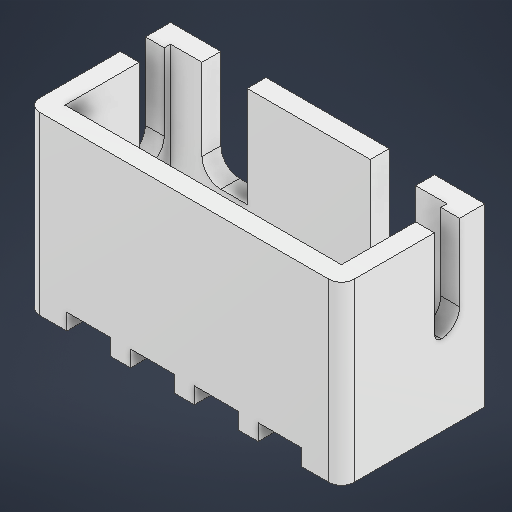
# Autodesk Inventor part: 4pin_head
Saved by Autodesk Inventor 2026 (Build 300175000, 175)
## iProperties
Created: 2025-04-18
Part Number: 4pin_head
Material: ABS Plastic
Document SubType Name: Modeling
Designer: ct_vi
Density: 1.06 g/cm^3
Appearance: Smooth - White
Author: ct_vi
Autodesk Inventor part; units mm, degrees
ref_plane "YZ Plane" through (0, 0, 0) normal (1, 0, 0) x (0, 1, 0)
ref_plane "XZ Plane" through (0, 0, 0) normal (0, 1, 0) x (-1, 0, 0)
ref_plane "XY Plane" through (0, 0, 0) normal (0, 0, 1) x (1, 0, 0)
sketch "Sketch1" plane through (0, 0, 0) normal (0, 1, 0) x (-1, 0, 0)
  line L0 (-10.6149, 17.6203) -> (28.5511, 17.6203) construction
  line L1 (28.5511, 17.6203) -> (28.5511, -21.5457) construction
  line L2 (28.5511, -21.5457) -> (-10.6149, -21.5457) construction
  line L3 (-10.6149, -21.5457) -> (-10.6149, 17.6203) construction
  line L4 (6.25, 2.85) -> (-6.25, 2.85)
  line L5 (-6.25, 2.85) -> (-6.25, -2.85)
  line L6 (-6.25, -2.85) -> (6.25, -2.85)
  line L7 (6.25, -2.85) -> (6.25, 2.85)
  line L8 (6.25, 2.85) -> (-6.25, -2.85) construction
  line L9 (-6.25, 2.85) -> (6.25, -2.85) construction
  line L10 (0, -2.85) -> (0, -0.85)
  line L11 (0, -0.85) -> (0, -0.54)
  line L12 (-0.96, -0.23) -> (-1.58, -0.23)
  line L13 (-1.58, -0.23) -> (-1.58, -0.85)
  line L14 (-1.58, -0.85) -> (-0.96, -0.85)
  line L15 (-0.96, -0.85) -> (-0.96, -0.23)
  line L16 (-0.96, -0.23) -> (-1.58, -0.85) construction
  line L17 (-1.58, -0.23) -> (-0.96, -0.85) construction
  line L18 (0.96, -0.23) -> (1.58, -0.23)
  line L19 (1.58, -0.23) -> (1.58, -0.85)
  line L20 (1.58, -0.85) -> (0.96, -0.85)
  line L21 (0.96, -0.85) -> (0.96, -0.23)
  line L22 (0.96, -0.23) -> (1.58, -0.85) construction
  line L23 (1.58, -0.23) -> (0.96, -0.85) construction
  line L24 (3.5, -0.23) -> (4.12, -0.23)
  line L25 (4.12, -0.23) -> (4.12, -0.85)
  line L26 (4.12, -0.85) -> (3.5, -0.85)
  line L27 (3.5, -0.85) -> (3.5, -0.23)
  line L28 (3.5, -0.23) -> (4.12, -0.85) construction
  line L29 (4.12, -0.23) -> (3.5, -0.85) construction
  line L30 (-3.5, -0.23) -> (-4.12, -0.23)
  line L31 (-4.12, -0.23) -> (-4.12, -0.85)
  line L32 (-4.12, -0.85) -> (-3.5, -0.85)
  line L33 (-3.5, -0.85) -> (-3.5, -0.23)
  line L34 (-3.5, -0.23) -> (-4.12, -0.85) construction
  line L35 (-4.12, -0.23) -> (-3.5, -0.85) construction
  line L36 (1.27, -0.54) -> (0, -0.54)
  line L37 (0, -0.54) -> (-1.27, -0.54)
  line L38 (-1.27, -0.54) -> (-3.81, -0.54)
  line L39 (-5.5, -2.1) -> (5.5, -2.1)
  line L40 (5.5, -2.1) -> (5.5, 2.1)
  line L41 (5.5, 2.1) -> (-5.5, 2.1)
  line L42 (-5.5, 2.1) -> (-5.5, -2.1)
  line L43 (-5.5, -2.1) -> (5.5, 2.1) construction
  line L44 (5.5, -2.1) -> (-5.5, 2.1) construction
  line L45 (0, -0.54) -> (0, -0.04)
  line L46 (-5.5, 0.2067) -> (5.5, 0.2067)
  line L47 (-5.5, -1.1747) -> (5.5, -1.1747)
  line L48 (5.5, -1.1747) -> (5.5, 0.2067)
  line L49 (-5.5, 0.2067) -> (-5.5, -1.1747)
  point P0 (0, 0)
  dimension "d11" = 12.5
  dimension "d12" = 5.7
  dimension "d43" = 2
  dimension "d44" = 0.31
  dimension "d57" = 0.62
  dimension "d58" = 0.62
  dimension "d59" = 2.54
  dimension "d66" = 11
  dimension "d68" = 0.75
  dimension "d72" = 0.5
  constraints: 92 end point, 14 parallel, 9 midpoint, 8 horizontal, 7 perpendicular, 3 point on line, 2 vertical, 2 other
  measures "d11" distance of L6.end L5.end
  measures "d12" distance of L5.end L4.end
  measures "d43" distance of L10.start L10.end
  measures "d44" distance of L10.end L11.end
  measures "d57" distance of L32.end L31.end
  measures "d58" distance of L31.end L30.end
  measures "d59" distance of L37.end L38.end
  measures "d66" distance of L41.end L40.end
  measures "d68" distance between parallel lines of L41 L4
  measures "d72" distance of L11.end L45.end
extrude "Extrusion1" add sketch "Sketch1" along normal blind 7 contours L7 L6 L5 L4
fillet "Fillet1" radius 0.5 2 edges at (6.25, 3.5, 2.85) (-6.25, 3.5, 2.85)
sketch "Sketch2" plane through (6.25, 0, -2.85) normal (0, 0, -1) x (-1, 0, 0)
  line L0 (-3.8851, 33.7763) -> (36.1854, 33.7763) construction
  line L1 (36.1854, 33.7763) -> (36.1854, -6.2941) construction
  line L2 (36.1854, -6.2941) -> (-3.8851, -6.2941) construction
  line L3 (-3.8851, -6.2941) -> (-3.8851, 33.7763) construction
  line L4 (6.25, 0) -> (6.25, 0.65)
  line L5 (0, 0) -> (12.5, 0) projected
  line L6 (5.85, 0) -> (6.65, 0)
  line L7 (6.25, 0.65) -> (3.71, 0.65)
  line L8 (3.71, 0.65) -> (4.11, 0.65)
  line L9 (4.11, 0.65) -> (3.31, 0.65)
  line L10 (3.31, 0.65) -> (3.31, 0)
  line L11 (3.31, 0) -> (4.11, 0)
  line L12 (4.11, 0) -> (4.11, 0.65)
  line L13 (6.25, 0.65) -> (8.79, 0.65)
  line L14 (8.79, 0.65) -> (8.39, 0.65)
  line L15 (8.39, 0.65) -> (9.19, 0.65)
  line L16 (9.19, 0.65) -> (9.19, 0)
  line L17 (9.19, 0) -> (8.39, 0)
  line L18 (8.39, 0) -> (8.39, 0.65)
  line L19 (6.25, 0.65) -> (6.65, 0.65)
  line L20 (6.65, 0.65) -> (5.85, 0.65)
  line L21 (5.85, 0.65) -> (5.85, 0)
  line L22 (5.85, 0) -> (6.65, 0)
  line L23 (6.65, 0) -> (6.65, 0.65)
  line L24 (9.19, 0.65) -> (10.93, 0.65)
  line L25 (10.93, 0.65) -> (10.93, 0)
  line L26 (10.93, 0.65) -> (12.5, 0.65)
  line L27 (3.31, 0.65) -> (1.57, 0.65)
  line L28 (1.57, 0.65) -> (1.57, 0)
  line L29 (0, 0) -> (0, 7)
  line L30 (0, 7) -> (2, 7)
  line L31 (2, 7) -> (2, 3)
  line L32 (12.5, 0) -> (12.5, 7)
  line L33 (12.5, 7) -> (10.5, 7)
  line L34 (10.5, 7) -> (10.5, 3)
  line L35 (2, 3) -> (3.8, 3)
  line L36 (3.8, 3) -> (3.8, 7)
  line L37 (3.8, 7) -> (2, 7)
  line L38 (10.5, 3) -> (8.7, 3)
  line L39 (8.7, 3) -> (8.7, 7)
  line L40 (8.7, 7) -> (10.5, 7)
  line L41 (1.57, 0.65) -> (0, 0.65)
  point P0 (6.65, 0.325)
  point P1 (8.79, 0.65)
  point P2 (3.71, 0.65)
  dimension "d112" = 0.65
  dimension "d114" = 0.8
  dimension "d122" = 2.54
  dimension "d123" = 0.4
  dimension "d124" = 0.8
  dimension "d125" = 2.54
  dimension "d126" = 0.4
  dimension "d127" = 0.8
  dimension "d128" = 0.4
  dimension "d129" = 0.8
  dimension "d130" = 1.74
  dimension "d131" = 1.74
  dimension "d132" = 1.74
  dimension "d136" = 7
  dimension "d137" = 2
  dimension "d138" = 4
  dimension "d139" = 2
  dimension "d140" = 4
  dimension "d141" = 1.8
  dimension "d142" = 1.8
  constraints: 74 end point, 14 perpendicular, 9 horizontal, 9 point on line, 6 parallel, 3 vertical, 1 midpoint, 2 other
  measures "d112" distance of L4.start L4.end
  measures "d114" distance of L6.end L6.start
  measures "d122" distance of L4.end L7.end
  measures "d123" distance of L7.end L8.end
  measures "d124" distance of L11.end L10.end
  measures "d125" distance of L4.end L13.end
  measures "d126" distance of L13.end L14.end
  measures "d127" distance of L16.end L17.end
  measures "d128" distance of L4.end L19.end
  measures "d129" distance of L22.end L6.start
  measures "d130" distance from line of L18 point (6.65, 0.325)
  measures "d131" distance of L15.end L24.end
  measures "d132" distance of L9.end L27.end
  measures "d136" distance of L5.start L29.end
  measures "d137" distance of L29.end L30.end
  measures "d138" distance of L30.end L31.end
  measures "d139" distance of L32.end L33.end
  measures "d140" distance of L33.end L34.end
  measures "d141" distance of L31.end L35.end
  measures "d142" distance of L34.end L38.end
extrude "Extrusion2" cut sketch "Sketch2" against normal through all contours L5 L12 L7 L21 | L23 L13 L18 L5 | L5 L28 L27 L10 | L16 L24 L25 L5
extrude "Extrusion3" cut sketch "Sketch2" against normal blind 0.75 contours L37 L36 L35 L31 | L34 L38 L39 L40
fillet "Fillet2" radius 0.75 2 edges at (4.25, 3, -2.475) (-4.25, 3, -2.475)
extrude "Extrusion4" add sketch "Sketch2" against normal through all contours L5 L21 L7 L4 | L4 L13 L23 L5 | L5 L10 L9 L7 L12 | L18 L13 L15 L16 L5 | L5 L29 L41 L28 | L25 L26 L32 L5
extrude "Extrusion5" add sketch "Sketch1" along normal blind 1 contours L47 L42 L46 L40
sketch "Sketch3" plane through (2.94, 0.65, -2.85) normal (0, -1, 0) x (1, 0, 0)
  line L0 (-9.19, 0) -> (-9.19, 5.2) projected
  line L1 (-9.19, 0) -> (3.31, 0)
  line L2 (3.31, 0) -> (3.31, 1.75)
  line L3 (3.31, 1.75) -> (-9.19, 1.75)
  line L4 (-9.19, 1.75) -> (-9.19, 0)
  point P0 (-2.94, 2.85)
  point P1 (-9.19, 1.75)
  dimension "d151" = 12.5
  dimension "d152" = 1.75
  constraints: 8 end point, 2 parallel, 1 horizontal, 1 perpendicular
  measures "d151" distance of L3.end L2.end
  measures "d152" distance of L2.end L1.end
extrude "Extrusion6" add sketch "Sketch3" against normal up to surface (0.35 mm away)
sketch "Sketch4" plane through (4.68, 0, -2.85) normal (-1, 0, 0) x (0, 0, 1)
  line L0 (1.6753, 0) -> (0, 0.65)
  line L1 (0, 0.65) -> (1.6753, 0.65) projected
  line L2 (0, 0.65) -> (1.6753, 0.65)
  line L3 (1.6753, 0.65) -> (1.6753, 0)
  point P0 (2.85, 0)
  constraints: 6 end point, 1 collinear, 1 perpendicular, 1 point on line
extrude "Extrusion7" add sketch "Sketch4" along normal blind 10
sketch "Sketch5" plane through (4.68, 0.65, 2.1) normal (0, 1, 0) x (1, 0, 0)
  line L0 (-10.18, 1.8933) -> (0.82, 1.8933) projected
  line L1 (0.82, 0) -> (-10.18, 0) projected
  line L2 (0.82, 1.8933) -> (-10.18, 1.8933)
  line L3 (-10.18, 1.8933) -> (-10.18, 0)
  line L4 (-10.18, 0) -> (0.82, 0)
  line L5 (0.82, 0) -> (0.82, 1.8933)
  point P0 (-4.68, 2.1)
  constraints: 8 end point, 2 parallel, 1 horizontal, 1 perpendicular
extrude "Extrusion8" add sketch "Sketch5" along normal blind 0.1
sketch "Sketch6" plane through (4.68, 0, 2.85) normal (-1, 0, 0) x (0, 0, 1)
  line L0 (-2.6433, 0.65) -> (0, 0.65)
  line L1 (0, 0.65) -> (-2.6433, 0)
  line L2 (-2.6433, 0) -> (-2.6433, 0.65)
  point P0 (-2.85, 0)
  constraints: 6 end point, 1 horizontal, 1 perpendicular
extrude "Extrusion9" add sketch "Sketch6" along normal up to surface (9.36 mm away)
sketch "Sketch8" plane through (-6.25, 0, -2.85) normal (-1, 0, 0) x (0, 0, 1)
  line L0 (22.0489, 31.2466) -> (22.0489, -8.2432) construction
  line L1 (22.0489, -8.2432) -> (-17.4409, -8.2432) construction
  line L2 (-17.4409, -8.2432) -> (-17.4409, 31.2466) construction
  line L3 (-17.4409, 31.2466) -> (22.0489, 31.2466) construction
  line L4 (0.75, 7) -> (0, 7) projected
  line L5 (0, 7) -> (1, 7)
  line L6 (1, 7) -> (2, 7)
  line L7 (2, 7) -> (2, 3.5)
  line L8 (1.7, 3.2) -> (1.75, 3.2)
  line L9 (1, 3.95) -> (1, 7)
  arc A0 (1, 3.95) -> (1.75, 3.2) centre (1.75, 3.95) ccw
  arc A1 (1.7, 3.2) -> (2, 3.5) centre (1.7, 3.5) ccw
  point P0 (2.85, 0)
  point P1 (2, 3.2)
  point P2 (1, 3.2)
  point P3 (1.7194, 3.2006)
  dimension "d211" = 1
  dimension "d212" = 1
  dimension "d213" = 3.8
  dimension "d216" = 0.3
  constraints: 10 end point, 4 point on circle, 4 point on line, 4 tangent, 2 centre point, 2 parallel, 1 collinear, 1 horizontal, 1 perpendicular, 2 other
  measures "d211" distance of L4.end L5.end
  measures "d212" distance of point (2, 3.2) point (1, 3.2)
  measures "d213" distance of L6.end point (2, 3.2)
  measures "d216" radius of A1
extrude "Extrusion10" cut sketch "Sketch8" against normal through all
body "Solid1"
